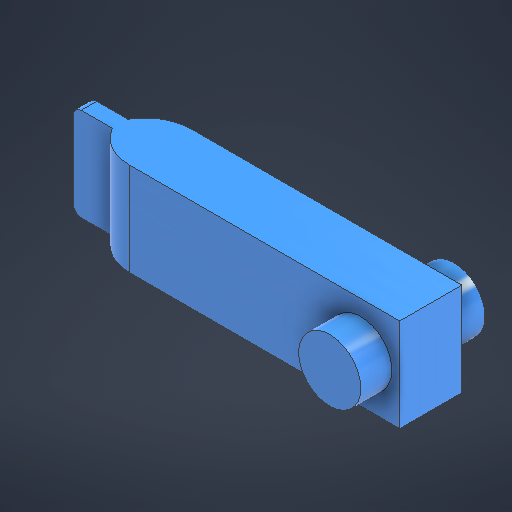
# Autodesk Inventor part: Part4final
Saved by Autodesk Inventor 2026 (Build 300175050, 175E)
## iProperties
Created: 2026-05-06
Part Number: Part4final
Material: Generic
Document SubType Name: Modeling
Designer: ptp527
Density: 1 g/cm^3
Appearance: Default
Author: ptp527
Autodesk Inventor part; units mm, degrees
ref_plane "YZ Plane" through (0, 0, 0) normal (1, 0, 0) x (0, 1, 0)
ref_plane "XZ Plane" through (0, 0, 0) normal (0, 1, 0) x (-1, 0, 0)
ref_plane "XY Plane" through (0, 0, 0) normal (0, 0, 1) x (1, 0, 0)
sketch "Sketch1" plane through (0, 0, 0) normal (0, 0, 1) x (1, 0, 0)
  line L0 (0, 0) -> (-200, 0)
  line L1 (-200, 0) -> (-200, 60)
  line L2 (-200, 60) -> (0, 60)
  line L3 (0, 60) -> (0, 0)
  dimension "d0" = 200
  dimension "d1" = 60
  constraints: 8 end point, 2 parallel, 1 horizontal, 1 perpendicular
  measures "d0" distance of L1.end L2.end
  measures "d1" distance of L0.end L1.end
extrude "Extrusion1" add sketch "Sketch1" along normal blind 40
sketch "Sketch2" plane through (0, 0, 40) normal (0, 0, 1) x (1, 0, 0)
  circle A0 centre (-25, 30) radius 20
  line L0 (0, 60) -> (-200, 60) projected
  line L1 (0, 0) -> (0, 60) projected
  dimension "d4" = 40
  dimension "d5" = 30
  dimension "d6" = 25
  constraints: 1 centre point
  measures "d4" diameter of A0
  measures "d5" distance from line of L0 A0.centre
  measures "d6" distance from line of L1 A0.centre
extrude "Extrusion2" add sketch "Sketch2" along normal mid plane 40
sketch "Sketch3" plane through (0, 0, 0) normal (0, 0, -1) x (-1, 0, 0)
  circle A0 centre (25, 30) radius 20 projected
  circle A1 centre (25, 30) radius 20
  point P0 (0, 0)
  constraints: 1 centre point, 1 coincident
extrude "Extrusion3" add sketch "Sketch3" along normal mid plane 40
sketch "Sketch4" plane through (-200, 0, 0) normal (-1, 0, 0) x (0, 0, 1)
  line L0 (0, 60) -> (40, 60) projected
  line L1 (25, 0) -> (15, 0)
  line L2 (15, 0) -> (15, 60)
  line L3 (15, 60) -> (25, 60)
  line L4 (25, 60) -> (25, 0)
  line L5 (0, 60) -> (0, 0) projected
  line L6 (40, 60) -> (40, 0) projected
  dimension "d11" = 10
  dimension "d12" = 60
  dimension "d13" = 15
  dimension "d14" = 15
  dimension "d15" = 60
  constraints: 8 end point, 2 parallel, 1 horizontal, 1 perpendicular, 1 point on line
  measures "d11" distance of L1.start L1.end
  measures "d12" distance of L3.end L1.start
  measures "d13" distance between parallel lines of L5 L2
  measures "d14" distance between parallel lines of L6 L4
  measures "d15" distance between parallel lines of L0 L1
extrude "Extrusion4" add sketch "Sketch4" along normal mid plane 50
fillet "Fillet1" radius 30 2 edges at (-200, 30, 0) (-200, 30, 40)
fillet "Fillet2" radius 5 2 edges at (-225, 60, 20) (-225, 0, 20)
body "Solid1"
